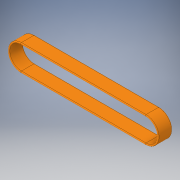
# Autodesk Inventor part: Polycord
Saved by Autodesk Inventor 2019 (Build 230136000, 136)
## iProperties
Created: 2018-11-03
Part Number: Polycord
Material: Rubber, Silicone
Document SubType Name: Modeling
Designer: woodk
Mass: 18.7524 g
Surface Area: 94.5004 cm^2
Volume: 15.0019 cm^3
Density: 1.25 g/cm^3
Appearance: Orange
Author: woodk
Autodesk Inventor part; units mm, degrees
ref_plane "YZ Plane" through (0, 0, 0) normal (1, 0, 0) x (0, 1, 0)
ref_plane "XZ Plane" through (0, 0, 0) normal (0, 1, 0) x (-1, 0, 0)
ref_plane "XY Plane" through (0, 0, 0) normal (0, 0, 1) x (1, 0, 0)
sketch "Sketch1" plane through (0, 0, 0) normal (0, 0, 1) x (1, 0, 0)
  line L0 (0, 0) -> (170.6562, 0)
  line L1 (170.6562, 33.7312) -> (0, 33.7312)
  arc A0 (0, 33.7312) -> (0, 0) centre (0, 16.8656) ccw
  arc A1 (170.6562, 0) -> (170.6562, 33.7312) centre (170.6562, 16.8656) ccw
  dimension "d2" = 16.8656
  dimension "d3" = 170.6562
  constraints: 4 end point, 4 point on circle, 4 vertical alignment, 2 centre point, 1 horizontal, 1 parallel
  measures "d2" radius of A1
  measures "d3" distance of A1.centre A0.centre
sketch "Sketch2" plane through (0, 0, 0) normal (1, 0, 0) x (0, 1, 0)
  arc A0 (0.9906, 0) -> (-0.9906, 0) centre (0, 0) ccw
  line L0 (-0.9906, 0) -> (0.9906, 0) construction
  line L1 (-0.9906, 0) -> (-0.9906, -17.0688)
  line L2 (0.9906, 0) -> (0.9906, -17.0688)
  arc A1 (-0.9906, -17.0688) -> (0.9906, -17.0688) centre (0, -17.0688) ccw
  dimension "d8" = 1.9812
  dimension "d9" = 19.05
  constraints: 6 end point, 4 point on circle, 2 centre point, 2 horizontal alignment, 2 tangent, 2 vertical, 1 coincident, 1 horizontal, 1 midpoint
  measures "d8" distance between parallel lines of L1 L2
sweep "Sweep1" add profiles "Sketch2" path "Sketch1"
body "Solid1"
